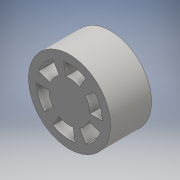
# Autodesk Inventor part: Flywheel Bracket
Saved by Autodesk Inventor 2016 (Build 200138000, 138)
## iProperties
Created: 2015-12-30
Part Number: Flywheel Bracket
Material: Generic
Document SubType Name: Modeling
Designer: jonathan
Density: 1 g/cm^3
Appearance: Default
Author: jonathan
Autodesk Inventor part; units mm, degrees
ref_plane "YZ Plane" through (0, 0, 0) normal (1, 0, 0) x (0, 1, 0)
ref_plane "XZ Plane" through (0, 0, 0) normal (0, 1, 0) x (-1, 0, 0)
ref_plane "XY Plane" through (0, 0, 0) normal (0, 0, 1) x (1, 0, 0)
sketch "Sketch1" plane through (0, 0, 0) normal (0, 1, 0) x (-1, 0, 0)
  circle A0 centre (0, 0) radius 10
  dimension "d0" = 20
  constraints: 1 centre point, 1 coincident
  measures "d0" diameter of A0
extrude "Extrusion1" add sketch "Sketch1" along normal blind 10
sketch "Sketch2" plane through (0, 10, 0) normal (0, 1, 0) x (1, 0, 0)
  line L0 (0, 0) -> (-9.4915, 0)
  arc A0 (-6.1284, 5.1423) -> (-8, 0) centre (0, 0) ccw
  arc A1 (-3.8302, 3.2139) -> (-5, 0) centre (0, 0) ccw
  line L1 (0, 0) -> (-3.8302, 3.2139)
  line L2 (-6.1284, 5.1423) -> (-3.8302, 3.2139)
  dimension "d3" = 40
  dimension "d4" = 5
  dimension "d5" = 8
  constraints: 6 end point, 4 point on circle, 2 centre point, 2 coincident, 2 point on line, 1 collinear, 1 horizontal
  measures "d3" angle of L0 L1
  measures "d4" radius of A1
  measures "d5" radius of A0
extrude "Extrusion2" cut sketch "Sketch2" against normal blind 10 contours L0 A0 L2 A1
pattern_circular "Circular Pattern1" count 6 over 360 about axis through (0, 10, 0) along (0, -1, 0) of "Extrusion2"
body "Solid1"
